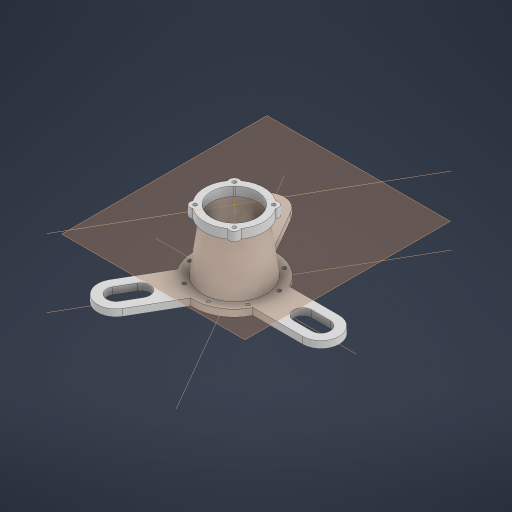
# Autodesk Inventor part: Część25
Saved by Autodesk Inventor 2023 (Build 270158000, 158)
## iProperties
Created: 2023-05-09
Part Number: Część25
Material: Ogólny
Document SubType Name: Modeling
Designer: Adam
Density: 1 g/cm^3
Appearance: Domyślna
Author: Adam
Autodesk Inventor part; units mm, degrees
ref_plane "YZ Plane" through (0, 0, 0) normal (1, 0, 0) x (0, 1, 0)
ref_plane "XZ Plane" through (0, 0, 0) normal (0, 1, 0) x (-1, 0, 0)
ref_plane "XY Plane" through (0, 0, 0) normal (0, 0, 1) x (1, 0, 0)
sketch "Szkic1" plane through (0, 0, 0) normal (0, 1, 0) x (-1, 0, 0)
  circle A0 centre (0, 0) radius 90
  dimension "d0" = 180
  constraints: 1 centre point, 1 coincident
  measures "d0" diameter of A0
extrude "Wyciągnięcie proste1" add sketch "Szkic1" along normal blind 15
sketch "Szkic2" plane through (0, 0, 0) normal (0, -1, 0) x (1, 0, 0)
  line L0 (70, 0) -> (190, 0) construction
  line L1 (70, -40) -> (190, -40)
  line L2 (190, 40) -> (70, 40)
  arc A0 (70, 40) -> (70, -40) centre (70, 0) ccw
  arc A1 (190, -40) -> (190, 40) centre (190, 0) ccw
  circle A2 centre (0, 0) radius 190
  arc A3 (-129.641, -144.5448) -> (-60.359, -184.5448) centre (-95, -164.5448) ccw
  line L3 (-60.359, -184.5448) -> (-0.359, -80.6218)
  line L4 (-69.641, -40.6218) -> (-129.641, -144.5448)
  arc A4 (-0.359, -80.6218) -> (-69.641, -40.6218) centre (-35, -60.6218) ccw
  arc A5 (-60.359, 184.5448) -> (-129.641, 144.5448) centre (-95, 164.5448) ccw
  line L5 (-129.641, 144.5448) -> (-69.641, 40.6218)
  line L6 (-0.359, 80.6218) -> (-60.359, 184.5448)
  arc A6 (-69.641, 40.6218) -> (-0.359, 80.6218) centre (-35, 60.6218) ccw
  point P0 (130, 0)
  point P1 (130, -40)
  point P2 (130, 40)
  point P3 (-30.359, -132.5833)
  point P4 (-99.641, -92.5833)
  point P5 (-99.641, 92.5833)
  point P6 (-30.359, 132.5833)
  dimension "d3" = 380
  dimension "d4" = 80
  dimension "d5" = 120
  dimension "d8" = 360
  constraints: 16 end point, 12 point on circle, 6 centre point, 4 tangent, 3 coincident, 3 midpoint, 1 horizontal, 1 horizontal alignment, 1 parallel, 40 other
  measures "d4" distance of point (130, -40) point (130, 40)
  measures "d5" distance of L2.start L2.end
extrude "Wyciągnięcie proste2" add sketch "Szkic2" against normal blind 15 contours A0 L2 A2 L1 | A2 L2 A1 L1 | L3 A3 L4 A2 | A2 L4 A4 L3 | L6 A6 L5 A2 | A2 L5 A5 L6
sketch "Szkic3" plane through (0, 0, 0) normal (0, -1, 0) x (1, 0, 0)
  arc A0 (190, -40) -> (190, 40) centre (190, 0) ccw projected
  line L0 (190, 0) -> (150, 0) construction
  line L1 (190, 20) -> (150, 20)
  line L2 (150, -20) -> (190, -20)
  arc A1 (190, -20) -> (190, 20) centre (190, 0) ccw
  arc A2 (150, 20) -> (150, -20) centre (150, 0) ccw
  line L3 (190, 40) -> (80.6226, 40) projected
  line L4 (80.6226, -40) -> (190, -40) projected
  point P0 (0, 0)
  point P1 (170, 0)
  dimension "d12" = 40
  constraints: 8 end point, 4 point on circle, 4 tangent, 3 parallel, 2 centre point, 1 horizontal, 1 midpoint
  measures "d12" diameter of A2
extrude "Wyciągnięcie proste3" cut sketch "Szkic3" against normal through all
sketch "Szkic4" plane through (0, 0, 0) normal (0, -1, 0) x (1, 0, 0)
  point P0 (0, 0)
  point P1 (0, 0)
  constraints: 1 coincident
pattern_circular "Szyk kołowy1" count 3 over 360 about axis through (0, 0, 0) along (0, -1, 0) of "Wyciągnięcie proste3"
sketch "Szkic5" plane through (0, 0, 0) normal (0, -1, 0) x (1, 0, 0)
  circle A0 centre (0, 0) radius 80
  point P0 (-40, 69.282)
  point P1 (-77.2741, 20.7055)
  point P2 (-69.282, -40)
  point P3 (-20.7055, -77.2741)
  point P4 (40, -69.282)
  point P5 (77.2741, -20.7055)
  point P6 (69.282, 40)
  point P7 (20.7055, 77.2741)
  dimension "d18" = 160
  dimension "d21" = 360
  constraints: 1 coincident, 12 other
hole "Otwór1" at (-40, 0, 69.282) at (20.7055, 0, 77.2741) at (69.282, 0, 40) at (77.2741, 0, -20.7055) at (40, 0, -69.282) at (-20.7055, 0, -77.2741) at (-69.282, 0, -40) at (-77.2741, 0, 20.7055) direction (0, 1, 0) diameter 8 end through all
sketch "Szkic6" plane through (0, 15, 0) normal (0, 1, 0) x (1, 0, 0)
  circle A0 centre (0, 0) radius 70
  dimension "d30" = 140
  constraints: 1 centre point, 1 coincident
  measures "d30" diameter of A0
ref_plane "Płaszczyzna konstrukcyjna1" through (0, 130, 0) normal (0, 1, 0) x (1, 0, 0)
sketch "Szkic7" plane through (0, 130, 0) normal (0, 1, 0) x (1, 0, 0)
  circle A0 centre (0, 0) radius 55
  dimension "d32" = 110
  constraints: 1 centre point, 1 coincident
  measures "d32" diameter of A0
loft "Wyciągnięcie złożone1" add profiles "Szkic6", "Szkic7"
sketch "Szkic8" plane through (0, 130, 0) normal (0, 1, 0) x (1, 0, 0)
  circle A0 centre (0, 0) radius 65
  dimension "d37" = 130
  constraints: 1 centre point, 1 coincident
  measures "d37" diameter of A0
extrude "Wyciągnięcie proste4" add sketch "Szkic8" along normal blind 20
sketch "Szkic9" plane through (0, 150, 0) normal (0, 1, 0) x (1, 0, 0)
  point P0 (0, 0)
sketch "Szkic11" plane through (0, 150, 0) normal (0, 1, 0) x (1, 0, 0)
  point P0 (0, 0)
sketch "Szkic12" plane through (0, 150, 0) normal (0, 1, 0) x (1, 0, 0)
  point P0 (0, 0)
sketch "Szkic13" plane through (0, 0, 0) normal (0, -1, 0) x (1, 0, 0)
  circle A0 centre (0, 0) radius 65
  dimension "d42" = 130
  constraints: 1 centre point, 1 coincident
  measures "d42" diameter of A0
extrude "Wyciągnięcie proste5" cut sketch "Szkic13" against normal blind 15
sketch "Szkic14" plane through (0, 15, 0) normal (0, -1, 0) x (1, 0, 0)
  point P0 (0, 0)
  point P1 (0, 0)
  constraints: 1 coincident
sketch "Szkic15" plane through (0, 130, 0) normal (0, 1, 0) x (1, 0, 0)
  circle A0 centre (0, 0) radius 50
  dimension "d45" = 100
  constraints: 1 centre point, 1 coincident
  measures "d45" diameter of A0
sketch "Szkic16" plane through (0, 150, 0) normal (0, 1, 0) x (1, 0, 0)
  circle A0 centre (0, 0) radius 50
  dimension "d46" = 100
  constraints: 1 centre point, 1 coincident
  measures "d46" diameter of A0
loft "Wyciągnięcie złożone2" cut profiles "Szkic15" section 1 edges at (-65, 15, 0)
extrude "Wyciągnięcie proste6" cut sketch "Szkic16" against normal through all
sketch "Szkic17" plane through (0, 150, 0) normal (0, 1, 0) x (1, 0, 0)
  point P0 (0, 0)
sketch "Szkic18" plane through (0, 150, 0) normal (0, 1, 0) x (1, 0, 0)
  line L0 (0, 0) -> (77.7817, 0) construction
  circle A0 centre (43, 43) radius 11
  circle A1 centre (0, 0) radius 50 projected
  line L1 (0, 0) -> (0, 77.7817) construction
  circle A2 centre (-43, 43) radius 11
  line L2 (0, 0) -> (-77.7817, 0) construction
  circle A3 centre (-43, -43) radius 11
  line L3 (0, 0) -> (0, -77.7817) construction
  circle A4 centre (43, -43) radius 11
  point P0 (-36.6324, -34.0304)
  point P1 (-34.0304, -36.6324)
  point P2 (34.0304, -36.6324)
  point P3 (36.6324, -34.0304)
  point P4 (34.0304, 36.6324)
  point P5 (36.6324, 34.0304)
  dimension "d54" = 22
  dimension "d55" = 43
  dimension "d58" = 360
  constraints: 8 end point, 4 centre point, 2 coincident, 1 horizontal, 19 other
  measures "d54" diameter of A0
  measures "d55" horizontal distance of A1.centre A0.centre
extrude "Wyciągnięcie proste7" add sketch "Szkic18" against normal blind 20 contours A0 A1 | A2 A1 | A1 A2 | A4 A1 | A1 A3 picked at (45.2627, 45.9315) picked at (45.2627, -45.9315) picked at (-45.1646, -46.0167)
sketch "Szkic19" plane through (0, 150, 0) normal (0, 1, 0) x (1, 0, 0)
  arc A0 (52.7718, 37.9491) -> (37.9491, 52.7718) centre (43, 43) ccw projected
  point P0 (0, 0)
  constraints: 1 coincident
hole "Otwór2" at (43, 150, -43) direction (0, -1, 0) diameter 8 depth 20 tip angle 118
pattern_circular "Szyk kołowy2" count 4 over 360 about axis through (0, 150, 0) along (0, 1, 0) of "Otwór2"
